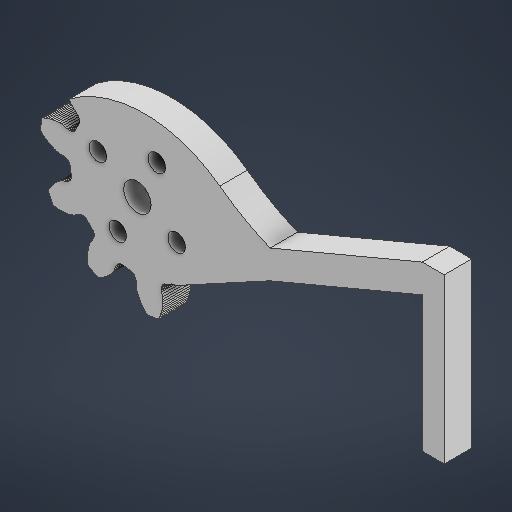
# Autodesk Inventor part: писюн
Saved by Autodesk Inventor 2025 (Build 290162000, 162)
## iProperties
Created: 2024-12-28
Part Number: писюн
Material: Типовые
Document SubType Name: Modeling
Designer: Phantom
Density: 1 g/cm^3
Appearance: По умолчанию
Author: Phantom
Autodesk Inventor part; units mm, degrees
(part 1 of 2)
ref_plane "YZ Plane" through (0, 0, 0) normal (1, 0, 0) x (0, 1, 0)
ref_plane "XZ Plane" through (0, 0, 0) normal (0, 1, 0) x (-1, 0, 0)
ref_plane "XY Plane" through (0, 0, 0) normal (0, 0, 1) x (1, 0, 0)
sketch "Эскиз1" plane through (0, 0, 0) normal (0, 0, 1) x (1, 0, 0)
  arc A0 (25.3405, 9.161) -> (8.4316, -5.5092) centre (48.8211, -34.9827) ccw
  arc A1 (16.1963, 14.3431) -> (25.3405, 9.161) centre (40.8164, 47.1281) ccw
  arc A2 (16.1963, 14.3431) -> (-11.1891, 14.3431) centre (2.5036, -3.8906) ccw
  line L0 (-11.1891, 14.3431) -> (-11.0924, 14.1698)
  line L1 (-11.0924, 14.1698) -> (-10.8798, 13.8428)
  line L2 (-10.8798, 13.8428) -> (-10.6476, 13.5415)
  line L3 (-10.6476, 13.5415) -> (-10.3902, 13.2744)
  line L4 (-10.3902, 13.2744) -> (-10.0964, 13.0589)
  line L5 (-10.0964, 13.0589) -> (-9.8198, 12.8188)
  line L6 (-9.8198, 12.8188) -> (-9.6918, 12.6838)
  line L7 (-9.6918, 12.6838) -> (-9.5723, 12.5363)
  line L8 (-9.5723, 12.5363) -> (-9.4633, 12.3731)
  line L9 (-9.4633, 12.3731) -> (-9.3681, 12.1883)
  line L10 (-9.3681, 12.1883) -> (-9.3278, 12.0845)
  line L11 (-9.3278, 12.0845) -> (-9.2943, 11.9695)
  line L12 (-9.2943, 11.9695) -> (-9.2712, 11.8376)
  line L13 (-9.2712, 11.8376) -> (-9.2668, 11.6743)
  line L14 (-9.2668, 11.6743) -> (-9.3696, 11.329)
  line L15 (-9.3696, 11.329) -> (-9.7265, 10.6764)
  line L16 (-9.7265, 10.6764) -> (-10.0432, 10.0032)
  line L17 (-10.0432, 10.0032) -> (-10.2615, 9.7167)
  line L18 (-10.2615, 9.7167) -> (-10.3959, 9.6239)
  line L19 (-10.3959, 9.6239) -> (-10.5161, 9.5649)
  line L20 (-10.5161, 9.5649) -> (-10.6287, 9.5241)
  line L21 (-10.6287, 9.5241) -> (-10.7364, 9.4955)
  line L22 (-10.7364, 9.4955) -> (-10.9417, 9.4634)
  line L23 (-10.9417, 9.4634) -> (-11.1379, 9.4552)
  line L24 (-11.1379, 9.4552) -> (-11.3274, 9.4648)
  line L25 (-11.3274, 9.4648) -> (-11.5119, 9.4885)
  line L26 (-11.5119, 9.4885) -> (-11.8689, 9.5704)
  line L27 (-11.8689, 9.5704) -> (-12.2162, 9.6807)
  line L28 (-12.2162, 9.6807) -> (-12.5837, 9.731)
  line L29 (-12.5837, 9.731) -> (-12.964, 9.741)
  line L30 (-12.964, 9.741) -> (-13.3534, 9.7199)
  line L31 (-13.3534, 9.7199) -> (-13.7498, 9.6714)
  line L32 (-13.7498, 9.6714) -> (-14.1519, 9.5976)
  line L33 (-14.1519, 9.5976) -> (-14.5586, 9.4998)
  line L34 (-14.5586, 9.4998) -> (-14.9687, 9.3787)
  line L35 (-14.9687, 9.3787) -> (-15.3815, 9.2349)
  line L36 (-15.3815, 9.2349) -> (-15.796, 9.069)
  line L37 (-15.796, 9.069) -> (-16.1075, 8.9301)
  line L38 (-16.1075, 8.9301) -> (-16.4414, 6.8067)
  line L39 (-16.4414, 6.8067) -> (-16.1875, 6.579)
  line L40 (-16.1875, 6.579) -> (-15.8439, 6.2938)
  line L41 (-15.8439, 6.2938) -> (-15.4952, 6.0303)
  line L42 (-15.4952, 6.0303) -> (-15.142, 5.7892)
  line L43 (-15.142, 5.7892) -> (-14.785, 5.5713)
  line L44 (-14.785, 5.5713) -> (-14.425, 5.3776)
  line L45 (-14.425, 5.3776) -> (-14.0625, 5.2099)
  line L46 (-14.0625, 5.2099) -> (-13.6984, 5.0703)
  line L47 (-13.6984, 5.0703) -> (-13.3334, 4.963)
  line L48 (-13.3334, 4.963) -> (-12.9682, 4.8982)
  line L49 (-12.9682, 4.8982) -> (-12.6038, 4.8965)
  line L50 (-12.6038, 4.8965) -> (-12.2389, 4.8649)
  line L51 (-12.2389, 4.8649) -> (-12.056, 4.8309)
  line L52 (-12.056, 4.8309) -> (-11.8727, 4.7818)
  line L53 (-11.8727, 4.7818) -> (-11.6885, 4.7139)
  line L54 (-11.6885, 4.7139) -> (-11.5029, 4.6203)
  line L55 (-11.5029, 4.6203) -> (-11.4093, 4.56)
  line L56 (-11.4093, 4.56) -> (-11.3146, 4.4866)
  line L57 (-11.3146, 4.4866) -> (-11.2183, 4.3936)
  line L58 (-11.2183, 4.3936) -> (-11.1188, 4.264)
  line L59 (-11.1188, 4.264) -> (-10.999, 3.9243)
  line L60 (-10.999, 3.9243) -> (-10.9042, 3.1865)
  line L61 (-10.9042, 3.1865) -> (-10.7647, 2.4558)
  line L62 (-10.7647, 2.4558) -> (-10.7729, 2.0956)
  line L63 (-10.7729, 2.0956) -> (-10.8272, 1.9416)
  line L64 (-10.8272, 1.9416) -> (-10.8897, 1.8232)
  line L65 (-10.8897, 1.8232) -> (-10.9568, 1.724)
  line L66 (-10.9568, 1.724) -> (-11.0271, 1.6375)
  line L67 (-11.0271, 1.6375) -> (-11.1743, 1.4909)
  line L68 (-11.1743, 1.4909) -> (-11.3282, 1.369)
  line L69 (-11.3282, 1.369) -> (-11.4872, 1.2653)
  line L70 (-11.4872, 1.2653) -> (-11.6504, 1.1761)
  line L71 (-11.6504, 1.1761) -> (-11.9874, 1.0325)
  line L72 (-11.9874, 1.0325) -> (-12.3332, 0.9175)
  line L73 (-12.3332, 0.9175) -> (-12.66, 0.7423)
  line L74 (-12.66, 0.7423) -> (-12.9736, 0.5268)
  line L75 (-12.9736, 0.5268) -> (-13.2762, 0.2808)
  line L76 (-13.2762, 0.2808) -> (-13.5684, 0.0086)
  line L77 (-13.5684, 0.0086) -> (-13.8504, -0.2874)
  line L78 (-13.8504, -0.2874) -> (-14.1218, -0.6056)
  line L79 (-14.1218, -0.6056) -> (-14.3824, -0.9447)
  line L80 (-14.3824, -0.9447) -> (-14.6319, -1.3036)
  line L81 (-14.6319, -1.3036) -> (-14.8697, -1.6815)
  line L82 (-14.8697, -1.6815) -> (-15.0401, -1.9769)
  line L83 (-15.0401, -1.9769) -> (-14.0621, -3.891)
  line L84 (-14.0621, -3.891) -> (-13.7228, -3.9261)
  line L85 (-13.7228, -3.9261) -> (-13.2773, -3.9548)
  line L86 (-13.2773, -3.9548) -> (-12.8403, -3.963)
  line L87 (-12.8403, -3.963) -> (-12.4128, -3.9505)
  line L88 (-12.4128, -3.9505) -> (-11.9959, -3.917)
  line L89 (-11.9959, -3.917) -> (-11.5908, -3.862)
  line L90 (-11.5908, -3.862) -> (-11.199, -3.7847)
  line L91 (-11.199, -3.7847) -> (-10.8224, -3.6836)
  line L92 (-10.8224, -3.6836) -> (-10.464, -3.5558)
  line L93 (-10.464, -3.5558) -> (-10.1304, -3.3936)
  line L94 (-10.1304, -3.3936) -> (-9.8347, -3.1808)
  line L95 (-9.8347, -3.1808) -> (-9.5209, -2.9918)
  line L96 (-9.5209, -2.9918) -> (-9.353, -2.9118)
  line L97 (-9.353, -2.9118) -> (-9.1758, -2.8438)
  line L98 (-9.1758, -2.8438) -> (-8.9868, -2.7905)
  line L99 (-8.9868, -2.7905) -> (-8.7817, -2.7571)
  line L100 (-8.7817, -2.7571) -> (-8.6705, -2.7509)
  line L101 (-8.6705, -2.7509) -> (-8.5508, -2.7546)
  line L102 (-8.5508, -2.7546) -> (-8.4182, -2.7733)
  line L103 (-8.4182, -2.7733) -> (-8.2615, -2.8196)
  line L104 (-8.2615, -2.8196) -> (-7.9649, -3.024)
  line L105 (-7.9649, -3.024) -> (-7.4545, -3.5652)
  line L106 (-7.4545, -3.5652) -> (-6.9122, -4.0744)
  line L107 (-6.9122, -4.0744) -> (-6.7071, -4.3705)
  line L108 (-6.7071, -4.3705) -> (-6.6604, -4.5271)
  line L109 (-6.6604, -4.5271) -> (-6.6415, -4.6596)
  line L110 (-6.6415, -4.6596) -> (-6.6374, -4.7793)
  line L111 (-6.6374, -4.7793) -> (-6.6435, -4.8906)
  line L112 (-6.6435, -4.8906) -> (-6.6764, -5.0958)
  line L113 (-6.6764, -5.0958) -> (-6.7292, -5.2848)
  line L114 (-6.7292, -5.2848) -> (-6.7969, -5.4622)
  line L115 (-6.7969, -5.4622) -> (-6.8765, -5.6303)
  line L116 (-6.8765, -5.6303) -> (-7.0647, -5.9445)
  line L117 (-7.0647, -5.9445) -> (-7.2769, -6.2407)
  line L118 (-7.2769, -6.2407) -> (-7.4384, -6.5746)
  line L119 (-7.4384, -6.5746) -> (-7.5654, -6.9333)
  line L120 (-7.5654, -6.9333) -> (-7.6656, -7.3102)
  line L121 (-7.6656, -7.3102) -> (-7.742, -7.7022)
  line L122 (-7.742, -7.7022) -> (-7.7961, -8.1074)
  line L123 (-7.7961, -8.1074) -> (-7.8287, -8.5243)
  line L124 (-7.8287, -8.5243) -> (-7.8403, -8.9518)
  line L125 (-7.8403, -8.9518) -> (-7.8311, -9.3888)
  line L126 (-7.8311, -9.3888) -> (-7.8013, -9.8343)
  line L127 (-7.8013, -9.8343) -> (-7.7656, -10.1735)
  line L128 (-7.7656, -10.1735) -> (-5.8492, -11.1472)
  line L129 (-5.8492, -11.1472) -> (-5.5542, -10.9761)
  line L130 (-5.5542, -10.9761) -> (-5.1768, -10.7375)
  line L131 (-5.1768, -10.7375) -> (-4.8185, -10.4872)
  line L132 (-4.8185, -10.4872) -> (-4.48, -10.2258)
  line L133 (-4.48, -10.2258) -> (-4.1624, -9.9537)
  line L134 (-4.1624, -9.9537) -> (-3.867, -9.6711)
  line L135 (-3.867, -9.6711) -> (-3.5955, -9.3782)
  line L136 (-3.5955, -9.3782) -> (-3.3502, -9.0751)
  line L137 (-3.3502, -9.0751) -> (-3.1354, -8.7611)
  line L138 (-3.1354, -8.7611) -> (-2.9609, -8.4338)
  line L139 (-2.9609, -8.4338) -> (-2.8467, -8.0877)
  line L140 (-2.8467, -8.0877) -> (-2.7039, -7.7505)
  line L141 (-2.7039, -7.7505) -> (-2.615, -7.5871)
  line L142 (-2.615, -7.5871) -> (-2.5117, -7.4278)
  line L143 (-2.5117, -7.4278) -> (-2.3901, -7.2737)
  line L144 (-2.3901, -7.2737) -> (-2.2438, -7.1261)
  line L145 (-2.2438, -7.1261) -> (-2.1575, -7.0556)
  line L146 (-2.1575, -7.0556) -> (-2.0585, -6.9883)
  line L147 (-2.0585, -6.9883) -> (-1.9402, -6.9255)
  line L148 (-1.9402, -6.9255) -> (-1.7863, -6.8709)
  line L149 (-1.7863, -6.8709) -> (-1.4262, -6.8619)
  line L150 (-1.4262, -6.8619) -> (-0.6951, -6.9997)
  line L151 (-0.6951, -6.9997) -> (0.0429, -7.0929)
  line L152 (0.0429, -7.0929) -> (0.3829, -7.2119)
  line L153 (0.3829, -7.2119) -> (0.5127, -7.3112)
  line L154 (0.5127, -7.3112) -> (0.6059, -7.4072)
  line L155 (0.6059, -7.4072) -> (0.6795, -7.5017)
  line L156 (0.6795, -7.5017) -> (0.74, -7.5953)
  line L157 (0.74, -7.5953) -> (0.834, -7.7806)
  line L158 (0.834, -7.7806) -> (0.9024, -7.9646)
  line L159 (0.9024, -7.9646) -> (0.9519, -8.1479)
  line L160 (0.9519, -8.1479) -> (0.9863, -8.3307)
  line L161 (0.9863, -8.3307) -> (1.0187, -8.6955)
  line L162 (1.0187, -8.6955) -> (1.0212, -9.0599)
  line L163 (1.0212, -9.0599) -> (1.0869, -9.4249)
  line L164 (1.0869, -9.4249) -> (1.1949, -9.7897)
  line L165 (1.1949, -9.7897) -> (1.3353, -10.1535)
  line L166 (1.3353, -10.1535) -> (1.5039, -10.5156)
  line L167 (1.5039, -10.5156) -> (1.6983, -10.8752)
  line L168 (1.6983, -10.8752) -> (1.9171, -11.2317)
  line L169 (1.9171, -11.2317) -> (2.159, -11.5843)
  line L170 (2.159, -11.5843) -> (2.4233, -11.9325)
  line L171 (2.4233, -11.9325) -> (2.7092, -12.2754)
  line L172 (2.7092, -12.2754) -> (2.9375, -12.5288)
  line L173 (2.9375, -12.5288) -> (5.0602, -12.1901)
  line L174 (5.0602, -12.1901) -> (5.1983, -11.8783)
  line L175 (5.1983, -11.8783) -> (5.3633, -11.4634)
  line L176 (5.3633, -11.4634) -> (5.5062, -11.0504)
  line L177 (5.5062, -11.0504) -> (5.6263, -10.6399)
  line L178 (5.6263, -10.6399) -> (5.7233, -10.2331)
  line L179 (5.7233, -10.2331) -> (5.7962, -9.8308)
  line L180 (5.7962, -9.8308) -> (5.8437, -9.4343)
  line L181 (5.8437, -9.4343) -> (5.864, -9.0449)
  line L182 (5.864, -9.0449) -> (5.8532, -8.6645)
  line L183 (5.8532, -8.6645) -> (5.802, -8.2972)
  line L184 (5.802, -8.2972) -> (5.691, -7.9502)
  line L185 (5.691, -7.9502) -> (5.6083, -7.5933)
  line L186 (5.6083, -7.5933) -> (5.5841, -7.4089)
  line L187 (5.5841, -7.4089) -> (5.5741, -7.2193)
  line L188 (5.5741, -7.2193) -> (5.5818, -7.0232)
  line L189 (5.5818, -7.0232) -> (5.6135, -6.8178)
  line L190 (5.6135, -6.8178) -> (5.6419, -6.7101)
  line L191 (5.6419, -6.7101) -> (5.6824, -6.5974)
  line L192 (5.6824, -6.5974) -> (5.7412, -6.4771)
  line L193 (5.7412, -6.4771) -> (5.8336, -6.3424)
  line L194 (5.8336, -6.3424) -> (6.1197, -6.1235)
  line L195 (6.1197, -6.1235) -> (6.7921, -5.8052)
  line L196 (6.7921, -5.8052) -> (7.444, -5.4468)
  line L197 (7.444, -5.4468) -> (7.789, -5.3433)
  line L198 (7.789, -5.3433) -> (7.9523, -5.3473)
  line L199 (7.9523, -5.3473) -> (8.0842, -5.3702)
  line L200 (8.0842, -5.3702) -> (8.1993, -5.4034)
  line L201 (8.1993, -5.4034) -> (8.3032, -5.4435)
  line L202 (8.3032, -5.4435) -> (8.4316, -5.5092)
  circle A3 centre (-5.9559, 8.675) radius 1.6
  circle A4 centre (-2.3455, -2.0471) radius 1.6
  circle A5 centre (8.3767, 1.5633) radius 1.6
  circle A6 centre (4.7663, 12.2855) radius 1.6
  circle A7 centre (1.2104, 5.1192) radius 2.5
  point P0 (0, 0)
  point P1 (-20.9679, -17.3277)
  constraints: 406 end point, 8 centre point, 6 point on circle
extrude "Выдавливание1" add sketch "Эскиз1" along normal blind 5
sketch "Эскиз2" plane through (0, 0, 0) normal (0, 0, -1) x (-1, 0, 0)
  line L0 (-8.3032, -5.4435) -> (-8.4316, -5.5092) projected
  line L1 (-8.4316, -5.5092) -> (-25.3405, -5.5092)
  line L2 (11.1891, 14.3431) -> (11.0924, 14.1698) projected
  arc A0 (11.1891, 14.3431) -> (-16.1963, 14.3431) centre (-2.5036, -3.8906) ccw projected
  arc A1 (-25.3405, 9.161) -> (-16.1963, 14.3431) centre (-40.8164, 47.1281) ccw projected
  arc A2 (-8.4316, -5.5092) -> (-25.3405, 9.161) centre (-48.8211, -34.9827) ccw projected
  line L3 (-8.3032, -5.4435) -> (-8.4316, -5.5092) projected
  line L4 (-8.1993, -5.4034) -> (-8.3032, -5.4435) projected
  line L5 (-8.0842, -5.3702) -> (-8.1993, -5.4034) projected
  line L6 (-7.9523, -5.3473) -> (-8.0842, -5.3702) projected
  line L7 (-7.789, -5.3433) -> (-7.9523, -5.3473) projected
  line L8 (-7.444, -5.4468) -> (-7.789, -5.3433) projected
  line L9 (-6.7921, -5.8052) -> (-7.444, -5.4468) projected
  line L10 (-6.1197, -6.1235) -> (-6.7921, -5.8052) projected
  line L11 (-5.8336, -6.3424) -> (-6.1197, -6.1235) projected
  line L12 (-5.7412, -6.4771) -> (-5.8336, -6.3424) projected
  line L13 (-5.6824, -6.5974) -> (-5.7412, -6.4771) projected
  line L14 (-5.6419, -6.7101) -> (-5.6824, -6.5974) projected
  line L15 (-5.6135, -6.8178) -> (-5.6419, -6.7101) projected
  line L16 (-5.5818, -7.0232) -> (-5.6135, -6.8178) projected
  line L17 (-5.5741, -7.2193) -> (-5.5818, -7.0232) projected
  line L18 (-5.5841, -7.4089) -> (-5.5741, -7.2193) projected
  line L19 (-5.6083, -7.5933) -> (-5.5841, -7.4089) projected
  line L20 (-5.691, -7.9502) -> (-5.6083, -7.5933) projected
  line L21 (-5.802, -8.2972) -> (-5.691, -7.9502) projected
  line L22 (-5.8532, -8.6645) -> (-5.802, -8.2972) projected
  line L23 (-5.864, -9.0449) -> (-5.8532, -8.6645) projected
  line L24 (-5.8437, -9.4343) -> (-5.864, -9.0449) projected
  line L25 (-5.7962, -9.8308) -> (-5.8437, -9.4343) projected
  line L26 (-5.7233, -10.2331) -> (-5.7962, -9.8308) projected
  line L27 (-5.6263, -10.6399) -> (-5.7233, -10.2331) projected
  line L28 (-5.5062, -11.0504) -> (-5.6263, -10.6399) projected
  line L29 (-5.3633, -11.4634) -> (-5.5062, -11.0504) projected
  line L30 (-5.1983, -11.8783) -> (-5.3633, -11.4634) projected
  line L31 (-5.0602, -12.1901) -> (-5.1983, -11.8783) projected
  line L32 (-2.9375, -12.5288) -> (-5.0602, -12.1901) projected
  line L33 (-2.7092, -12.2754) -> (-2.9375, -12.5288) projected
  line L34 (-2.4233, -11.9325) -> (-2.7092, -12.2754) projected
  line L35 (-2.159, -11.5843) -> (-2.4233, -11.9325) projected
  line L36 (-1.9171, -11.2317) -> (-2.159, -11.5843) projected
  line L37 (-1.6983, -10.8752) -> (-1.9171, -11.2317) projected
  line L38 (-1.5039, -10.5156) -> (-1.6983, -10.8752) projected
  line L39 (-1.3353, -10.1535) -> (-1.5039, -10.5156) projected
  line L40 (-1.1949, -9.7897) -> (-1.3353, -10.1535) projected
  line L41 (-1.0869, -9.4249) -> (-1.1949, -9.7897) projected
  line L42 (-1.0212, -9.0599) -> (-1.0869, -9.4249) projected
  line L43 (-1.0187, -8.6955) -> (-1.0212, -9.0599) projected
  line L44 (-0.9863, -8.3307) -> (-1.0187, -8.6955) projected
  line L45 (-0.9519, -8.1479) -> (-0.9863, -8.3307) projected
  line L46 (-0.9024, -7.9646) -> (-0.9519, -8.1479) projected
  line L47 (-0.834, -7.7806) -> (-0.9024, -7.9646) projected
  line L48 (-0.74, -7.5953) -> (-0.834, -7.7806) projected
  line L49 (-0.6795, -7.5017) -> (-0.74, -7.5953) projected
  line L50 (-0.6059, -7.4072) -> (-0.6795, -7.5017) projected
  line L51 (-0.5127, -7.3112) -> (-0.6059, -7.4072) projected
  line L52 (-0.3829, -7.2119) -> (-0.5127, -7.3112) projected
  line L53 (-0.0429, -7.0929) -> (-0.3829, -7.2119) projected
  line L54 (0.6951, -6.9997) -> (-0.0429, -7.0929) projected
  line L55 (1.4262, -6.8619) -> (0.6951, -6.9997) projected
  line L56 (1.7863, -6.8709) -> (1.4262, -6.8619) projected
  line L57 (1.9402, -6.9255) -> (1.7863, -6.8709) projected
  line L58 (2.0585, -6.9883) -> (1.9402, -6.9255) projected
  line L59 (2.1575, -7.0556) -> (2.0585, -6.9883) projected
  line L60 (2.2438, -7.1261) -> (2.1575, -7.0556) projected
  line L61 (2.3901, -7.2737) -> (2.2438, -7.1261) projected
  line L62 (2.5117, -7.4278) -> (2.3901, -7.2737) projected
  line L63 (2.615, -7.5871) -> (2.5117, -7.4278) projected
  line L64 (2.7039, -7.7505) -> (2.615, -7.5871) projected
  line L65 (2.8467, -8.0877) -> (2.7039, -7.7505) projected
  line L66 (2.9609, -8.4338) -> (2.8467, -8.0877) projected
  line L67 (3.1354, -8.7611) -> (2.9609, -8.4338) projected
  line L68 (3.3502, -9.0751) -> (3.1354, -8.7611) projected
  line L69 (3.5955, -9.3782) -> (3.3502, -9.0751) projected
  line L70 (3.867, -9.6711) -> (3.5955, -9.3782) projected
  line L71 (4.1624, -9.9537) -> (3.867, -9.6711) projected
  line L72 (4.48, -10.2258) -> (4.1624, -9.9537) projected
  line L73 (4.8185, -10.4872) -> (4.48, -10.2258) projected
  line L74 (5.1768, -10.7375) -> (4.8185, -10.4872) projected
  line L75 (5.5542, -10.9761) -> (5.1768, -10.7375) projected
  line L76 (5.8492, -11.1472) -> (5.5542, -10.9761) projected
  line L77 (7.7656, -10.1735) -> (5.8492, -11.1472) projected
  line L78 (7.8013, -9.8343) -> (7.7656, -10.1735) projected
  line L79 (7.8311, -9.3888) -> (7.8013, -9.8343) projected
  line L80 (7.8403, -8.9518) -> (7.8311, -9.3888) projected
  line L81 (7.8287, -8.5243) -> (7.8403, -8.9518) projected
  line L82 (7.7961, -8.1074) -> (7.8287, -8.5243) projected
  line L83 (7.742, -7.7022) -> (7.7961, -8.1074) projected
  line L84 (7.6656, -7.3102) -> (7.742, -7.7022) projected
  line L85 (7.5654, -6.9333) -> (7.6656, -7.3102) projected
  line L86 (7.4384, -6.5746) -> (7.5654, -6.9333) projected
  line L87 (7.2769, -6.2407) -> (7.4384, -6.5746) projected
  line L88 (7.0647, -5.9445) -> (7.2769, -6.2407) projected
  line L89 (6.8765, -5.6303) -> (7.0647, -5.9445) projected
  line L90 (6.7969, -5.4622) -> (6.8765, -5.6303) projected
  line L91 (6.7292, -5.2848) -> (6.7969, -5.4622) projected
  line L92 (6.6764, -5.0958) -> (6.7292, -5.2848) projected
  line L93 (6.6435, -4.8906) -> (6.6764, -5.0958) projected
  line L94 (6.6374, -4.7793) -> (6.6435, -4.8906) projected
  line L95 (6.6415, -4.6596) -> (6.6374, -4.7793) projected
  line L96 (6.6604, -4.5271) -> (6.6415, -4.6596) projected
  line L97 (6.7071, -4.3705) -> (6.6604, -4.5271) projected
  line L98 (6.9122, -4.0744) -> (6.7071, -4.3705) projected
  line L99 (7.4545, -3.5652) -> (6.9122, -4.0744) projected
  line L100 (7.9649, -3.024) -> (7.4545, -3.5652) projected
  line L101 (8.2615, -2.8196) -> (7.9649, -3.024) projected
  line L102 (8.4182, -2.7733) -> (8.2615, -2.8196) projected
  line L103 (8.5508, -2.7546) -> (8.4182, -2.7733) projected
  line L104 (8.6705, -2.7509) -> (8.5508, -2.7546) projected
  line L105 (8.7817, -2.7571) -> (8.6705, -2.7509) projected
  line L106 (8.9868, -2.7905) -> (8.7817, -2.7571) projected
  line L107 (9.1758, -2.8438) -> (8.9868, -2.7905) projected
  line L108 (9.353, -2.9118) -> (9.1758, -2.8438) projected
  line L109 (9.5209, -2.9918) -> (9.353, -2.9118) projected
  line L110 (9.8347, -3.1808) -> (9.5209, -2.9918) projected
  line L111 (10.1304, -3.3936) -> (9.8347, -3.1808) projected
  line L112 (10.464, -3.5558) -> (10.1304, -3.3936) projected
  line L113 (10.8224, -3.6836) -> (10.464, -3.5558) projected
  line L114 (11.199, -3.7847) -> (10.8224, -3.6836) projected
  line L115 (11.5908, -3.862) -> (11.199, -3.7847) projected
  line L116 (11.9959, -3.917) -> (11.5908, -3.862) projected
  line L117 (12.4128, -3.9505) -> (11.9959, -3.917) projected
  line L118 (12.8403, -3.963) -> (12.4128, -3.9505) projected
  line L119 (13.2773, -3.9548) -> (12.8403, -3.963) projected
  line L120 (13.7228, -3.9261) -> (13.2773, -3.9548) projected
  line L121 (14.0621, -3.891) -> (13.7228, -3.9261) projected
  line L122 (15.0401, -1.9769) -> (14.0621, -3.891) projected
  line L123 (14.8697, -1.6815) -> (15.0401, -1.9769) projected
  line L124 (14.6319, -1.3036) -> (14.8697, -1.6815) projected
  line L125 (14.3824, -0.9447) -> (14.6319, -1.3036) projected
  line L126 (14.1218, -0.6056) -> (14.3824, -0.9447) projected
  line L127 (13.8504, -0.2874) -> (14.1218, -0.6056) projected
  line L128 (13.5684, 0.0086) -> (13.8504, -0.2874) projected
  line L129 (13.2762, 0.2808) -> (13.5684, 0.0086) projected
  line L130 (12.9736, 0.5268) -> (13.2762, 0.2808) projected
  line L131 (12.66, 0.7423) -> (12.9736, 0.5268) projected
  line L132 (12.3332, 0.9175) -> (12.66, 0.7423) projected
  line L133 (11.9874, 1.0325) -> (12.3332, 0.9175) projected
  line L134 (11.6504, 1.1761) -> (11.9874, 1.0325) projected
  line L135 (11.4872, 1.2653) -> (11.6504, 1.1761) projected
  line L136 (11.3282, 1.369) -> (11.4872, 1.2653) projected
  line L137 (11.1743, 1.4909) -> (11.3282, 1.369) projected
  line L138 (11.0271, 1.6375) -> (11.1743, 1.4909) projected
  line L139 (10.9568, 1.724) -> (11.0271, 1.6375) projected
  line L140 (10.8897, 1.8232) -> (10.9568, 1.724) projected
  line L141 (10.8272, 1.9416) -> (10.8897, 1.8232) projected
  line L142 (10.7729, 2.0956) -> (10.8272, 1.9416) projected
  line L143 (10.7647, 2.4558) -> (10.7729, 2.0956) projected
  line L144 (10.9042, 3.1865) -> (10.7647, 2.4558) projected
  line L145 (10.999, 3.9243) -> (10.9042, 3.1865) projected
  line L146 (11.1188, 4.264) -> (10.999, 3.9243) projected
  line L147 (11.2183, 4.3936) -> (11.1188, 4.264) projected
  line L148 (11.3146, 4.4866) -> (11.2183, 4.3936) projected
  line L149 (11.4093, 4.56) -> (11.3146, 4.4866) projected
  line L150 (11.5029, 4.6203) -> (11.4093, 4.56) projected
  line L151 (11.6885, 4.7139) -> (11.5029, 4.6203) projected
  line L152 (11.8727, 4.7818) -> (11.6885, 4.7139) projected
  line L153 (12.056, 4.8309) -> (11.8727, 4.7818) projected
  line L154 (12.2389, 4.8649) -> (12.056, 4.8309) projected
  line L155 (12.6038, 4.8965) -> (12.2389, 4.8649) projected
  line L156 (12.9682, 4.8982) -> (12.6038, 4.8965) projected
  line L157 (13.3334, 4.963) -> (12.9682, 4.8982) projected
  line L158 (13.6984, 5.0703) -> (13.3334, 4.963) projected
  line L159 (14.0625, 5.2099) -> (13.6984, 5.0703) projected
  line L160 (14.425, 5.3776) -> (14.0625, 5.2099) projected
  line L161 (14.785, 5.5713) -> (14.425, 5.3776) projected
  line L162 (15.142, 5.7892) -> (14.785, 5.5713) projected
  line L163 (15.4952, 6.0303) -> (15.142, 5.7892) projected
  line L164 (15.8439, 6.2938) -> (15.4952, 6.0303) projected
  line L165 (16.1875, 6.579) -> (15.8439, 6.2938) projected
  line L166 (16.4414, 6.8067) -> (16.1875, 6.579) projected
  line L167 (16.1075, 8.9301) -> (16.4414, 6.8067) projected
  line L168 (15.796, 9.069) -> (16.1075, 8.9301) projected
  line L169 (15.3815, 9.2349) -> (15.796, 9.069) projected
  line L170 (14.9687, 9.3787) -> (15.3815, 9.2349) projected
  line L171 (14.5586, 9.4998) -> (14.9687, 9.3787) projected
  line L172 (14.1519, 9.5976) -> (14.5586, 9.4998) projected
  line L173 (13.7498, 9.6714) -> (14.1519, 9.5976) projected
  line L174 (13.3534, 9.7199) -> (13.7498, 9.6714) projected
  line L175 (12.964, 9.741) -> (13.3534, 9.7199) projected
  line L176 (12.5837, 9.731) -> (12.964, 9.741) projected
  line L177 (12.2162, 9.6807) -> (12.5837, 9.731) projected
  line L178 (11.8689, 9.5704) -> (12.2162, 9.6807) projected
  line L179 (11.5119, 9.4885) -> (11.8689, 9.5704) projected
  line L180 (11.3274, 9.4648) -> (11.5119, 9.4885) projected
  line L181 (11.1379, 9.4552) -> (11.3274, 9.4648) projected
  line L182 (10.9417, 9.4634) -> (11.1379, 9.4552) projected
  line L183 (10.7364, 9.4955) -> (10.9417, 9.4634) projected
  line L184 (10.6287, 9.5241) -> (10.7364, 9.4955) projected
  line L185 (10.5161, 9.5649) -> (10.6287, 9.5241) projected
  line L186 (10.3959, 9.6239) -> (10.5161, 9.5649) projected
  line L187 (10.2615, 9.7167) -> (10.3959, 9.6239) projected
  line L188 (10.0432, 10.0032) -> (10.2615, 9.7167) projected
  line L189 (9.7265, 10.6764) -> (10.0432, 10.0032) projected
  line L190 (9.3696, 11.329) -> (9.7265, 10.6764) projected
  line L191 (9.2668, 11.6743) -> (9.3696, 11.329) projected
  line L192 (9.2712, 11.8376) -> (9.2668, 11.6743) projected
  line L193 (9.2943, 11.9695) -> (9.2712, 11.8376) projected
  line L194 (9.3278, 12.0845) -> (9.2943, 11.9695) projected
  line L195 (9.3681, 12.1883) -> (9.3278, 12.0845) projected
  line L196 (9.4633, 12.3731) -> (9.3681, 12.1883) projected
  line L197 (9.5723, 12.5363) -> (9.4633, 12.3731) projected
  line L198 (9.6918, 12.6838) -> (9.5723, 12.5363) projected
  line L199 (9.8198, 12.8188) -> (9.6918, 12.6838) projected
  line L200 (10.0964, 13.0589) -> (9.8198, 12.8188) projected
  line L201 (10.3902, 13.2744) -> (10.0964, 13.0589) projected
  line L202 (10.6476, 13.5415) -> (10.3902, 13.2744) projected
  line L203 (10.8798, 13.8428) -> (10.6476, 13.5415) projected
  line L204 (11.0924, 14.1698) -> (10.8798, 13.8428) projected
  circle A3 centre (-8.3767, 1.5633) radius 1.6 projected
  circle A4 centre (2.3455, -2.0471) radius 1.6 projected
  circle A5 centre (5.9559, 8.675) radius 1.6 projected
  circle A6 centre (-4.7663, 12.2855) radius 1.6 projected
  circle A7 centre (-1.2104, 5.1192) radius 2.5 projected
  line L205 (-25.3405, 9.161) -> (-25.3405, -5.5092)
  point P0 (0, 0)
  constraints: 4 end point, 1 horizontal, 1 perpendicular
extrude "Выдавливание2" add sketch "Эскиз2" against normal up to surface (5 mm away) contours L1 L205 A2
sketch "Эскиз3" plane through (0, 0, 0) normal (0, 0, -1) x (-1, 0, 0)
  line L0 (-25.3405, 9.161) -> (-25.3405, -5.5092) projected
  line L1 (-25.3405, 9.161) -> (-53, 20.778)
  line L2 (-53, 20.778) -> (-76.2555, 1.8259)
  line L3 (-76.2555, 1.8259) -> (-73.7286, -1.2748)
  line L4 (-73.7286, -1.2748) -> (-53, 15.6179)
  line L5 (-53, 15.6179) -> (-25.3405, 4.0009)
  line L6 (11.1891, 14.3431) -> (11.0924, 14.1698) projected
  arc A0 (11.1891, 14.3431) -> (-16.1963, 14.3431) centre (-2.5036, -3.8906) ccw projected
  arc A1 (-25.3405, 9.161) -> (-16.1963, 14.3431) centre (-40.8164, 47.1281) ccw projected
  line L7 (-25.3405, 9.161) -> (-25.3405, -5.5092) projected
  line L8 (-25.3405, -5.5092) -> (-8.4316, -5.5092) projected
  line L9 (-8.3032, -5.4435) -> (-8.4316, -5.5092) projected
  line L10 (-8.1993, -5.4034) -> (-8.3032, -5.4435) projected
  line L11 (-8.0842, -5.3702) -> (-8.1993, -5.4034) projected
  line L12 (-7.9523, -5.3473) -> (-8.0842, -5.3702) projected
  line L13 (-7.789, -5.3433) -> (-7.9523, -5.3473) projected
  line L14 (-7.444, -5.4468) -> (-7.789, -5.3433) projected
  line L15 (-6.7921, -5.8052) -> (-7.444, -5.4468) projected
  line L16 (-6.1197, -6.1235) -> (-6.7921, -5.8052) projected
  line L17 (-5.8336, -6.3424) -> (-6.1197, -6.1235) projected
  line L18 (-5.7412, -6.4771) -> (-5.8336, -6.3424) projected
  line L19 (-5.6824, -6.5974) -> (-5.7412, -6.4771) projected
  line L20 (-5.6419, -6.7101) -> (-5.6824, -6.5974) projected
  line L21 (-5.6135, -6.8178) -> (-5.6419, -6.7101) projected
  line L22 (-5.5818, -7.0232) -> (-5.6135, -6.8178) projected
  line L23 (-5.5741, -7.2193) -> (-5.5818, -7.0232) projected
  line L24 (-5.5841, -7.4089) -> (-5.5741, -7.2193) projected
  line L25 (-5.6083, -7.5933) -> (-5.5841, -7.4089) projected
  line L26 (-5.691, -7.9502) -> (-5.6083, -7.5933) projected
  line L27 (-5.802, -8.2972) -> (-5.691, -7.9502) projected
  line L28 (-5.8532, -8.6645) -> (-5.802, -8.2972) projected
  line L29 (-5.864, -9.0449) -> (-5.8532, -8.6645) projected
  line L30 (-5.8437, -9.4343) -> (-5.864, -9.0449) projected
  line L31 (-5.7962, -9.8308) -> (-5.8437, -9.4343) projected
  line L32 (-5.7233, -10.2331) -> (-5.7962, -9.8308) projected
  line L33 (-5.6263, -10.6399) -> (-5.7233, -10.2331) projected
  line L34 (-5.5062, -11.0504) -> (-5.6263, -10.6399) projected
  line L35 (-5.3633, -11.4634) -> (-5.5062, -11.0504) projected
  line L36 (-5.1983, -11.8783) -> (-5.3633, -11.4634) projected
  line L37 (-5.0602, -12.1901) -> (-5.1983, -11.8783) projected
  line L38 (-2.9375, -12.5288) -> (-5.0602, -12.1901) projected
  line L39 (-2.7092, -12.2754) -> (-2.9375, -12.5288) projected
  line L40 (-2.4233, -11.9325) -> (-2.7092, -12.2754) projected
  line L41 (-2.159, -11.5843) -> (-2.4233, -11.9325) projected
  line L42 (-1.9171, -11.2317) -> (-2.159, -11.5843) projected
  line L43 (-1.6983, -10.8752) -> (-1.9171, -11.2317) projected
  line L44 (-1.5039, -10.5156) -> (-1.6983, -10.8752) projected
  line L45 (-1.3353, -10.1535) -> (-1.5039, -10.5156) projected
  line L46 (-1.1949, -9.7897) -> (-1.3353, -10.1535) projected
  line L47 (-1.0869, -9.4249) -> (-1.1949, -9.7897) projected
  line L48 (-1.0212, -9.0599) -> (-1.0869, -9.4249) projected
  line L49 (-1.0187, -8.6955) -> (-1.0212, -9.0599) projected
  line L50 (-0.9863, -8.3307) -> (-1.0187, -8.6955) projected
  line L51 (-0.9519, -8.1479) -> (-0.9863, -8.3307) projected
  line L52 (-0.9024, -7.9646) -> (-0.9519, -8.1479) projected
  line L53 (-0.834, -7.7806) -> (-0.9024, -7.9646) projected
  line L54 (-0.74, -7.5953) -> (-0.834, -7.7806) projected
  line L55 (-0.6795, -7.5017) -> (-0.74, -7.5953) projected
  line L56 (-0.6059, -7.4072) -> (-0.6795, -7.5017) projected
  line L57 (-0.5127, -7.3112) -> (-0.6059, -7.4072) projected
  line L58 (-0.3829, -7.2119) -> (-0.5127, -7.3112) projected
  line L59 (-0.0429, -7.0929) -> (-0.3829, -7.2119) projected
  line L60 (0.6951, -6.9997) -> (-0.0429, -7.0929) projected
  line L61 (1.4262, -6.8619) -> (0.6951, -6.9997) projected
  line L62 (1.7863, -6.8709) -> (1.4262, -6.8619) projected
  line L63 (1.9402, -6.9255) -> (1.7863, -6.8709) projected
  line L64 (2.0585, -6.9883) -> (1.9402, -6.9255) projected
  line L65 (2.1575, -7.0556) -> (2.0585, -6.9883) projected
  line L66 (2.2438, -7.1261) -> (2.1575, -7.0556) projected
  line L67 (2.3901, -7.2737) -> (2.2438, -7.1261) projected
  line L68 (2.5117, -7.4278) -> (2.3901, -7.2737) projected
  line L69 (2.615, -7.5871) -> (2.5117, -7.4278) projected
  line L70 (2.7039, -7.7505) -> (2.615, -7.5871) projected
  line L71 (2.8467, -8.0877) -> (2.7039, -7.7505) projected
  line L72 (2.9609, -8.4338) -> (2.8467, -8.0877) projected
  line L73 (3.1354, -8.7611) -> (2.9609, -8.4338) projected
  line L74 (3.3502, -9.0751) -> (3.1354, -8.7611) projected
  line L75 (3.5955, -9.3782) -> (3.3502, -9.0751) projected
  line L76 (3.867, -9.6711) -> (3.5955, -9.3782) projected
  line L77 (4.1624, -9.9537) -> (3.867, -9.6711) projected
  line L78 (4.48, -10.2258) -> (4.1624, -9.9537) projected
  line L79 (4.8185, -10.4872) -> (4.48, -10.2258) projected
  line L80 (5.1768, -10.7375) -> (4.8185, -10.4872) projected
  line L81 (5.5542, -10.9761) -> (5.1768, -10.7375) projected
  line L82 (5.8492, -11.1472) -> (5.5542, -10.9761) projected
  line L83 (7.7656, -10.1735) -> (5.8492, -11.1472) projected
  line L84 (7.8013, -9.8343) -> (7.7656, -10.1735) projected
  line L85 (7.8311, -9.3888) -> (7.8013, -9.8343) projected
  line L86 (7.8403, -8.9518) -> (7.8311, -9.3888) projected
  line L87 (7.8287, -8.5243) -> (7.8403, -8.9518) projected
  line L88 (7.7961, -8.1074) -> (7.8287, -8.5243) projected
  line L89 (7.742, -7.7022) -> (7.7961, -8.1074) projected
  line L90 (7.6656, -7.3102) -> (7.742, -7.7022) projected
  line L91 (7.5654, -6.9333) -> (7.6656, -7.3102) projected
  line L92 (7.4384, -6.5746) -> (7.5654, -6.9333) projected
  line L93 (7.2769, -6.2407) -> (7.4384, -6.5746) projected
  line L94 (7.0647, -5.9445) -> (7.2769, -6.2407) projected
  line L95 (6.8765, -5.6303) -> (7.0647, -5.9445) projected
  line L96 (6.7969, -5.4622) -> (6.8765, -5.6303) projected
  line L97 (6.7292, -5.2848) -> (6.7969, -5.4622) projected
  line L98 (6.6764, -5.0958) -> (6.7292, -5.2848) projected
  line L99 (6.6435, -4.8906) -> (6.6764, -5.0958) projected
  line L100 (6.6374, -4.7793) -> (6.6435, -4.8906) projected
  line L101 (6.6415, -4.6596) -> (6.6374, -4.7793) projected
  line L102 (6.6604, -4.5271) -> (6.6415, -4.6596) projected
  line L103 (6.7071, -4.3705) -> (6.6604, -4.5271) projected
  line L104 (6.9122, -4.0744) -> (6.7071, -4.3705) projected
  line L105 (7.4545, -3.5652) -> (6.9122, -4.0744) projected
  line L106 (7.9649, -3.024) -> (7.4545, -3.5652) projected
  line L107 (8.2615, -2.8196) -> (7.9649, -3.024) projected
  line L108 (8.4182, -2.7733) -> (8.2615, -2.8196) projected
  line L109 (8.5508, -2.7546) -> (8.4182, -2.7733) projected
  line L110 (8.6705, -2.7509) -> (8.5508, -2.7546) projected
  line L111 (8.7817, -2.7571) -> (8.6705, -2.7509) projected
  line L112 (8.9868, -2.7905) -> (8.7817, -2.7571) projected
  line L113 (9.1758, -2.8438) -> (8.9868, -2.7905) projected
  line L114 (9.353, -2.9118) -> (9.1758, -2.8438) projected
  line L115 (9.5209, -2.9918) -> (9.353, -2.9118) projected
  line L116 (9.8347, -3.1808) -> (9.5209, -2.9918) projected
  line L117 (10.1304, -3.3936) -> (9.8347, -3.1808) projected
  line L118 (10.464, -3.5558) -> (10.1304, -3.3936) projected
  line L119 (10.8224, -3.6836) -> (10.464, -3.5558) projected
  line L120 (11.199, -3.7847) -> (10.8224, -3.6836) projected
  line L121 (11.5908, -3.862) -> (11.199, -3.7847) projected
  line L122 (11.9959, -3.917) -> (11.5908, -3.862) projected
  line L123 (12.4128, -3.9505) -> (11.9959, -3.917) projected
  line L124 (12.8403, -3.963) -> (12.4128, -3.9505) projected
  line L125 (13.2773, -3.9548) -> (12.8403, -3.963) projected
  line L126 (13.7228, -3.9261) -> (13.2773, -3.9548) projected
  line L127 (14.0621, -3.891) -> (13.7228, -3.9261) projected
  line L128 (15.0401, -1.9769) -> (14.0621, -3.891) projected
  line L129 (14.8697, -1.6815) -> (15.0401, -1.9769) projected
  line L130 (14.6319, -1.3036) -> (14.8697, -1.6815) projected
  line L131 (14.3824, -0.9447) -> (14.6319, -1.3036) projected
  line L132 (14.1218, -0.6056) -> (14.3824, -0.9447) projected
  line L133 (13.8504, -0.2874) -> (14.1218, -0.6056) projected
  line L134 (13.5684, 0.0086) -> (13.8504, -0.2874) projected
  line L135 (13.2762, 0.2808) -> (13.5684, 0.0086) projected
  line L136 (12.9736, 0.5268) -> (13.2762, 0.2808) projected
  line L137 (12.66, 0.7423) -> (12.9736, 0.5268) projected
  line L138 (12.3332, 0.9175) -> (12.66, 0.7423) projected
  line L139 (11.9874, 1.0325) -> (12.3332, 0.9175) projected
  line L140 (11.6504, 1.1761) -> (11.9874, 1.0325) projected
  line L141 (11.4872, 1.2653) -> (11.6504, 1.1761) projected
  line L142 (11.3282, 1.369) -> (11.4872, 1.2653) projected
  line L143 (11.1743, 1.4909) -> (11.3282, 1.369) projected
  line L144 (11.0271, 1.6375) -> (11.1743, 1.4909) projected
  line L145 (10.9568, 1.724) -> (11.0271, 1.6375) projected
  line L146 (10.8897, 1.8232) -> (10.9568, 1.724) projected
  line L147 (10.8272, 1.9416) -> (10.8897, 1.8232) projected
  line L148 (10.7729, 2.0956) -> (10.8272, 1.9416) projected
  line L149 (10.7647, 2.4558) -> (10.7729, 2.0956) projected
  line L150 (10.9042, 3.1865) -> (10.7647, 2.4558) projected
  line L151 (10.999, 3.9243) -> (10.9042, 3.1865) projected
  line L152 (11.1188, 4.264) -> (10.999, 3.9243) projected
  line L153 (11.2183, 4.3936) -> (11.1188, 4.264) projected
  line L154 (11.3146, 4.4866) -> (11.2183, 4.3936) projected
  line L155 (11.4093, 4.56) -> (11.3146, 4.4866) projected
  line L156 (11.5029, 4.6203) -> (11.4093, 4.56) projected
  line L157 (11.6885, 4.7139) -> (11.5029, 4.6203) projected
  line L158 (11.8727, 4.7818) -> (11.6885, 4.7139) projected
  line L159 (12.056, 4.8309) -> (11.8727, 4.7818) projected
  line L160 (12.2389, 4.8649) -> (12.056, 4.8309) projected
  line L161 (12.6038, 4.8965) -> (12.2389, 4.8649) projected
  line L162 (12.9682, 4.8982) -> (12.6038, 4.8965) projected
  line L163 (13.3334, 4.963) -> (12.9682, 4.8982) projected
  line L164 (13.6984, 5.0703) -> (13.3334, 4.963) projected
  line L165 (14.0625, 5.2099) -> (13.6984, 5.0703) projected
  line L166 (14.425, 5.3776) -> (14.0625, 5.2099) projected
  line L167 (14.785, 5.5713) -> (14.425, 5.3776) projected
  line L168 (15.142, 5.7892) -> (14.785, 5.5713) projected
  line L169 (15.4952, 6.0303) -> (15.142, 5.7892) projected
  line L170 (15.8439, 6.2938) -> (15.4952, 6.0303) projected
  line L171 (16.1875, 6.579) -> (15.8439, 6.2938) projected
  line L172 (16.4414, 6.8067) -> (16.1875, 6.579) projected
  line L173 (16.1075, 8.9301) -> (16.4414, 6.8067) projected
  line L174 (15.796, 9.069) -> (16.1075, 8.9301) projected
  line L175 (15.3815, 9.2349) -> (15.796, 9.069) projected
  line L176 (14.9687, 9.3787) -> (15.3815, 9.2349) projected
  line L177 (14.5586, 9.4998) -> (14.9687, 9.3787) projected
  line L178 (14.1519, 9.5976) -> (14.5586, 9.4998) projected
  line L179 (13.7498, 9.6714) -> (14.1519, 9.5976) projected
  line L180 (13.3534, 9.7199) -> (13.7498, 9.6714) projected
  line L181 (12.964, 9.741) -> (13.3534, 9.7199) projected
  line L182 (12.5837, 9.731) -> (12.964, 9.741) projected
  line L183 (12.2162, 9.6807) -> (12.5837, 9.731) projected
  line L184 (11.8689, 9.5704) -> (12.2162, 9.6807) projected
  line L185 (11.5119, 9.4885) -> (11.8689, 9.5704) projected
  line L186 (11.3274, 9.4648) -> (11.5119, 9.4885) projected
  line L187 (11.1379, 9.4552) -> (11.3274, 9.4648) projected
  line L188 (10.9417, 9.4634) -> (11.1379, 9.4552) projected
  line L189 (10.7364, 9.4955) -> (10.9417, 9.4634) projected
  line L190 (10.6287, 9.5241) -> (10.7364, 9.4955) projected
  line L191 (10.5161, 9.5649) -> (10.6287, 9.5241) projected
  line L192 (10.3959, 9.6239) -> (10.5161, 9.5649) projected
  line L193 (10.2615, 9.7167) -> (10.3959, 9.6239) projected
  line L194 (10.0432, 10.0032) -> (10.2615, 9.7167) projected
  line L195 (9.7265, 10.6764) -> (10.0432, 10.0032) projected
  line L196 (9.3696, 11.329) -> (9.7265, 10.6764) projected
  line L197 (9.2668, 11.6743) -> (9.3696, 11.329) projected
  line L198 (9.2712, 11.8376) -> (9.2668, 11.6743) projected
  line L199 (9.2943, 11.9695) -> (9.2712, 11.8376) projected
  line L200 (9.3278, 12.0845) -> (9.2943, 11.9695) projected
  line L201 (9.3681, 12.1883) -> (9.3278, 12.0845) projected
  line L202 (9.4633, 12.3731) -> (9.3681, 12.1883) projected
  line L203 (9.5723, 12.5363) -> (9.4633, 12.3731) projected
  line L204 (9.6918, 12.6838) -> (9.5723, 12.5363) projected
  line L205 (9.8198, 12.8188) -> (9.6918, 12.6838) projected
  line L206 (10.0964, 13.0589) -> (9.8198, 12.8188) projected
  line L207 (10.3902, 13.2744) -> (10.0964, 13.0589) projected
  line L208 (10.6476, 13.5415) -> (10.3902, 13.2744) projected
  line L209 (10.8798, 13.8428) -> (10.6476, 13.5415) projected
  line L210 (11.0924, 14.1698) -> (10.8798, 13.8428) projected
  circle A2 centre (-8.3767, 1.5633) radius 1.6 projected
  circle A3 centre (2.3455, -2.0471) radius 1.6 projected
  circle A4 centre (5.9559, 8.675) radius 1.6 projected
  circle A5 centre (-4.7663, 12.2855) radius 1.6 projected
  circle A6 centre (-1.2104, 5.1192) radius 2.5 projected
  point P0 (0, 0)
  dimension "d4" = 30
  dimension "d5" = 30
  dimension "d6" = 4
  constraints: 10 end point, 2 perpendicular, 1 parallel, 1 point on line
  measures "d4" distance of L0.start L1.end
  measures "d5" distance of L1.end L2.end
  measures "d6" distance of L2.end L3.end
extrude "Выдавливание3" add sketch "Эскиз3" against normal up to surface (5 mm away) contours L0 L5 L4 L3 L2 L1
sketch "Эскиз4" plane through (0, 0, 0) normal (0, 0, -1) x (-1, 0, 0)
  line L0 (11.1891, 14.3431) -> (11.0924, 14.1698) projected
  arc A0 (11.1891, 14.3431) -> (-16.1963, 14.3431) centre (-2.5036, -3.8906) ccw projected
  arc A1 (-25.3405, 9.161) -> (-16.1963, 14.3431) centre (-40.8164, 47.1281) ccw projected
  line L1 (-25.3405, 9.161) -> (-53, 20.778) projected
  line L2 (-53, 20.778) -> (-76.2555, 1.8259) projected
  line L3 (-76.2555, 1.8259) -> (-73.7286, -1.2748) projected
  line L4 (-73.7286, -1.2748) -> (-53, 15.6179) projected
  line L5 (-53, 15.6179) -> (-25.3405, 4.0009) projected
  line L6 (-25.3405, 4.0009) -> (-25.3405, -5.5092) projected
  line L7 (-25.3405, -5.5092) -> (-8.4316, -5.5092) projected
  line L8 (-8.3032, -5.4435) -> (-8.4316, -5.5092) projected
  line L9 (-8.1993, -5.4034) -> (-8.3032, -5.4435) projected
  line L10 (-8.0842, -5.3702) -> (-8.1993, -5.4034) projected
  line L11 (-7.9523, -5.3473) -> (-8.0842, -5.3702) projected
  line L12 (-7.789, -5.3433) -> (-7.9523, -5.3473) projected
  line L13 (-7.444, -5.4468) -> (-7.789, -5.3433) projected
  line L14 (-6.7921, -5.8052) -> (-7.444, -5.4468) projected
  line L15 (-6.1197, -6.1235) -> (-6.7921, -5.8052) projected
  line L16 (-5.8336, -6.3424) -> (-6.1197, -6.1235) projected
  line L17 (-5.7412, -6.4771) -> (-5.8336, -6.3424) projected
  line L18 (-5.6824, -6.5974) -> (-5.7412, -6.4771) projected
  line L19 (-5.6419, -6.7101) -> (-5.6824, -6.5974) projected
  line L20 (-5.6135, -6.8178) -> (-5.6419, -6.7101) projected
  line L21 (-5.5818, -7.0232) -> (-5.6135, -6.8178) projected
  line L22 (-5.5741, -7.2193) -> (-5.5818, -7.0232) projected
  line L23 (-5.5841, -7.4089) -> (-5.5741, -7.2193) projected
  line L24 (-5.6083, -7.5933) -> (-5.5841, -7.4089) projected
  line L25 (-5.691, -7.9502) -> (-5.6083, -7.5933) projected
  line L26 (-5.802, -8.2972) -> (-5.691, -7.9502) projected
  line L27 (-5.8532, -8.6645) -> (-5.802, -8.2972) projected
  line L28 (-5.864, -9.0449) -> (-5.8532, -8.6645) projected
  line L29 (-5.8437, -9.4343) -> (-5.864, -9.0449) projected
  line L30 (-5.7962, -9.8308) -> (-5.8437, -9.4343) projected
  line L31 (-5.7233, -10.2331) -> (-5.7962, -9.8308) projected
  line L32 (-5.6263, -10.6399) -> (-5.7233, -10.2331) projected
  line L33 (-5.5062, -11.0504) -> (-5.6263, -10.6399) projected
  line L34 (-5.3633, -11.4634) -> (-5.5062, -11.0504) projected
  line L35 (-5.1983, -11.8783) -> (-5.3633, -11.4634) projected
  line L36 (-5.0602, -12.1901) -> (-5.1983, -11.8783) projected
  line L37 (-2.9375, -12.5288) -> (-5.0602, -12.1901) projected
  line L38 (-2.7092, -12.2754) -> (-2.9375, -12.5288) projected
  line L39 (-2.4233, -11.9325) -> (-2.7092, -12.2754) projected
  line L40 (-2.159, -11.5843) -> (-2.4233, -11.9325) projected
  line L41 (-1.9171, -11.2317) -> (-2.159, -11.5843) projected
  line L42 (-1.6983, -10.8752) -> (-1.9171, -11.2317) projected
  line L43 (-1.5039, -10.5156) -> (-1.6983, -10.8752) projected
  line L44 (-1.3353, -10.1535) -> (-1.5039, -10.5156) projected
  line L45 (-1.1949, -9.7897) -> (-1.3353, -10.1535) projected
  line L46 (-1.0869, -9.4249) -> (-1.1949, -9.7897) projected
  line L47 (-1.0212, -9.0599) -> (-1.0869, -9.4249) projected
  line L48 (-1.0187, -8.6955) -> (-1.0212, -9.0599) projected
  line L49 (-0.9863, -8.3307) -> (-1.0187, -8.6955) projected
  line L50 (-0.9519, -8.1479) -> (-0.9863, -8.3307) projected
  line L51 (-0.9024, -7.9646) -> (-0.9519, -8.1479) projected
  line L52 (-0.834, -7.7806) -> (-0.9024, -7.9646) projected
  line L53 (-0.74, -7.5953) -> (-0.834, -7.7806) projected
  line L54 (-0.6795, -7.5017) -> (-0.74, -7.5953) projected
  line L55 (-0.6059, -7.4072) -> (-0.6795, -7.5017) projected
  line L56 (-0.5127, -7.3112) -> (-0.6059, -7.4072) projected
  line L57 (-0.3829, -7.2119) -> (-0.5127, -7.3112) projected
  line L58 (-0.0429, -7.0929) -> (-0.3829, -7.2119) projected
  line L59 (0.6951, -6.9997) -> (-0.0429, -7.0929) projected
  line L60 (1.4262, -6.8619) -> (0.6951, -6.9997) projected
  line L61 (1.7863, -6.8709) -> (1.4262, -6.8619) projected
  line L62 (1.9402, -6.9255) -> (1.7863, -6.8709) projected
  line L63 (2.0585, -6.9883) -> (1.9402, -6.9255) projected
  line L64 (2.1575, -7.0556) -> (2.0585, -6.9883) projected
  line L65 (2.2438, -7.1261) -> (2.1575, -7.0556) projected
  line L66 (2.3901, -7.2737) -> (2.2438, -7.1261) projected
  line L67 (2.5117, -7.4278) -> (2.3901, -7.2737) projected
  line L68 (2.615, -7.5871) -> (2.5117, -7.4278) projected
  line L69 (2.7039, -7.7505) -> (2.615, -7.5871) projected
  line L70 (2.8467, -8.0877) -> (2.7039, -7.7505) projected
  line L71 (2.9609, -8.4338) -> (2.8467, -8.0877) projected
  line L72 (3.1354, -8.7611) -> (2.9609, -8.4338) projected
  line L73 (3.3502, -9.0751) -> (3.1354, -8.7611) projected
  line L74 (3.5955, -9.3782) -> (3.3502, -9.0751) projected
  line L75 (3.867, -9.6711) -> (3.5955, -9.3782) projected
  line L76 (4.1624, -9.9537) -> (3.867, -9.6711) projected
  line L77 (4.48, -10.2258) -> (4.1624, -9.9537) projected
  line L78 (4.8185, -10.4872) -> (4.48, -10.2258) projected
  line L79 (5.1768, -10.7375) -> (4.8185, -10.4872) projected
  line L80 (5.5542, -10.9761) -> (5.1768, -10.7375) projected
  line L81 (5.8492, -11.1472) -> (5.5542, -10.9761) projected
  line L82 (7.7656, -10.1735) -> (5.8492, -11.1472) projected
  line L83 (7.8013, -9.8343) -> (7.7656, -10.1735) projected
  line L84 (7.8311, -9.3888) -> (7.8013, -9.8343) projected
  line L85 (7.8403, -8.9518) -> (7.8311, -9.3888) projected
  line L86 (7.8287, -8.5243) -> (7.8403, -8.9518) projected
  line L87 (7.7961, -8.1074) -> (7.8287, -8.5243) projected
  line L88 (7.742, -7.7022) -> (7.7961, -8.1074) projected
  line L89 (7.6656, -7.3102) -> (7.742, -7.7022) projected
  line L90 (7.5654, -6.9333) -> (7.6656, -7.3102) projected
  line L91 (7.4384, -6.5746) -> (7.5654, -6.9333) projected
  line L92 (7.2769, -6.2407) -> (7.4384, -6.5746) projected
  line L93 (7.0647, -5.9445) -> (7.2769, -6.2407) projected
  line L94 (6.8765, -5.6303) -> (7.0647, -5.9445) projected
  line L95 (6.7969, -5.4622) -> (6.8765, -5.6303) projected
  line L96 (6.7292, -5.2848) -> (6.7969, -5.4622) projected
  line L97 (6.6764, -5.0958) -> (6.7292, -5.2848) projected
  line L98 (6.6435, -4.8906) -> (6.6764, -5.0958) projected
  line L99 (6.6374, -4.7793) -> (6.6435, -4.8906) projected
  line L100 (6.6415, -4.6596) -> (6.6374, -4.7793) projected
  line L101 (6.6604, -4.5271) -> (6.6415, -4.6596) projected
  line L102 (6.7071, -4.3705) -> (6.6604, -4.5271) projected
  line L103 (6.9122, -4.0744) -> (6.7071, -4.3705) projected
  line L104 (7.4545, -3.5652) -> (6.9122, -4.0744) projected
  line L105 (7.9649, -3.024) -> (7.4545, -3.5652) projected
  line L106 (8.2615, -2.8196) -> (7.9649, -3.024) projected
  line L107 (8.4182, -2.7733) -> (8.2615, -2.8196) projected
  line L108 (8.5508, -2.7546) -> (8.4182, -2.7733) projected
  line L109 (8.6705, -2.7509) -> (8.5508, -2.7546) projected
  line L110 (8.7817, -2.7571) -> (8.6705, -2.7509) projected
  line L111 (8.9868, -2.7905) -> (8.7817, -2.7571) projected
  line L112 (9.1758, -2.8438) -> (8.9868, -2.7905) projected
  line L113 (9.353, -2.9118) -> (9.1758, -2.8438) projected
  line L114 (9.5209, -2.9918) -> (9.353, -2.9118) projected
  line L115 (9.8347, -3.1808) -> (9.5209, -2.9918) projected
  line L116 (10.1304, -3.3936) -> (9.8347, -3.1808) projected
  line L117 (10.464, -3.5558) -> (10.1304, -3.3936) projected
  line L118 (10.8224, -3.6836) -> (10.464, -3.5558) projected
  line L119 (11.199, -3.7847) -> (10.8224, -3.6836) projected
  line L120 (11.5908, -3.862) -> (11.199, -3.7847) projected
  line L121 (11.9959, -3.917) -> (11.5908, -3.862) projected
  line L122 (12.4128, -3.9505) -> (11.9959, -3.917) projected
  line L123 (12.8403, -3.963) -> (12.4128, -3.9505) projected
  line L124 (13.2773, -3.9548) -> (12.8403, -3.963) projected
  line L125 (13.7228, -3.9261) -> (13.2773, -3.9548) projected
  line L126 (14.0621, -3.891) -> (13.7228, -3.9261) projected
  line L127 (15.0401, -1.9769) -> (14.0621, -3.891) projected
  line L128 (14.8697, -1.6815) -> (15.0401, -1.9769) projected
  line L129 (14.6319, -1.3036) -> (14.8697, -1.6815) projected
  line L130 (14.3824, -0.9447) -> (14.6319, -1.3036) projected
  line L131 (14.1218, -0.6056) -> (14.3824, -0.9447) projected
  line L132 (13.8504, -0.2874) -> (14.1218, -0.6056) projected
  line L133 (13.5684, 0.0086) -> (13.8504, -0.2874) projected
  line L134 (13.2762, 0.2808) -> (13.5684, 0.0086) projected
  line L135 (12.9736, 0.5268) -> (13.2762, 0.2808) projected
  line L136 (12.66, 0.7423) -> (12.9736, 0.5268) projected
  line L137 (12.3332, 0.9175) -> (12.66, 0.7423) projected
  line L138 (11.9874, 1.0325) -> (12.3332, 0.9175) projected
  line L139 (11.6504, 1.1761) -> (11.9874, 1.0325) projected
  line L140 (11.4872, 1.2653) -> (11.6504, 1.1761) projected
  line L141 (11.3282, 1.369) -> (11.4872, 1.2653) projected
  line L142 (11.1743, 1.4909) -> (11.3282, 1.369) projected
  line L143 (11.0271, 1.6375) -> (11.1743, 1.4909) projected
  line L144 (10.9568, 1.724) -> (11.0271, 1.6375) projected
  line L145 (10.8897, 1.8232) -> (10.9568, 1.724) projected
  line L146 (10.8272, 1.9416) -> (10.8897, 1.8232) projected
  line L147 (10.7729, 2.0956) -> (10.8272, 1.9416) projected
  line L148 (10.7647, 2.4558) -> (10.7729, 2.0956) projected
  line L149 (10.9042, 3.1865) -> (10.7647, 2.4558) projected
  line L150 (10.999, 3.9243) -> (10.9042, 3.1865) projected
  line L151 (11.1188, 4.264) -> (10.999, 3.9243) projected
  line L152 (11.2183, 4.3936) -> (11.1188, 4.264) projected
  line L153 (11.3146, 4.4866) -> (11.2183, 4.3936) projected
  line L154 (11.4093, 4.56) -> (11.3146, 4.4866) projected
  line L155 (11.5029, 4.6203) -> (11.4093, 4.56) projected
  line L156 (11.6885, 4.7139) -> (11.5029, 4.6203) projected
  line L157 (11.8727, 4.7818) -> (11.6885, 4.7139) projected
  line L158 (12.056, 4.8309) -> (11.8727, 4.7818) projected
  line L159 (12.2389, 4.8649) -> (12.056, 4.8309) projected
  line L160 (12.6038, 4.8965) -> (12.2389, 4.8649) projected
  line L161 (12.9682, 4.8982) -> (12.6038, 4.8965) projected
  line L162 (13.3334, 4.963) -> (12.9682, 4.8982) projected
  line L163 (13.6984, 5.0703) -> (13.3334, 4.963) projected
  line L164 (14.0625, 5.2099) -> (13.6984, 5.0703) projected
  line L165 (14.425, 5.3776) -> (14.0625, 5.2099) projected
  line L166 (14.785, 5.5713) -> (14.425, 5.3776) projected
  line L167 (15.142, 5.7892) -> (14.785, 5.5713) projected
  line L168 (15.4952, 6.0303) -> (15.142, 5.7892) projected
  line L169 (15.8439, 6.2938) -> (15.4952, 6.0303) projected
  line L170 (16.1875, 6.579) -> (15.8439, 6.2938) projected
  line L171 (16.4414, 6.8067) -> (16.1875, 6.579) projected
  line L172 (16.1075, 8.9301) -> (16.4414, 6.8067) projected
  line L173 (15.796, 9.069) -> (16.1075, 8.9301) projected
  line L174 (15.3815, 9.2349) -> (15.796, 9.069) projected
  line L175 (14.9687, 9.3787) -> (15.3815, 9.2349) projected
  line L176 (14.5586, 9.4998) -> (14.9687, 9.3787) projected
  line L177 (14.1519, 9.5976) -> (14.5586, 9.4998) projected
  line L178 (13.7498, 9.6714) -> (14.1519, 9.5976) projected
  line L179 (13.3534, 9.7199) -> (13.7498, 9.6714) projected
  line L180 (12.964, 9.741) -> (13.3534, 9.7199) projected
  line L181 (12.5837, 9.731) -> (12.964, 9.741) projected
  line L182 (12.2162, 9.6807) -> (12.5837, 9.731) projected
  line L183 (11.8689, 9.5704) -> (12.2162, 9.6807) projected
  line L184 (11.5119, 9.4885) -> (11.8689, 9.5704) projected
  line L185 (11.3274, 9.4648) -> (11.5119, 9.4885) projected
  line L186 (11.1379, 9.4552) -> (11.3274, 9.4648) projected
  line L187 (10.9417, 9.4634) -> (11.1379, 9.4552) projected
  line L188 (10.7364, 9.4955) -> (10.9417, 9.4634) projected
  line L189 (10.6287, 9.5241) -> (10.7364, 9.4955) projected
  line L190 (10.5161, 9.5649) -> (10.6287, 9.5241) projected
  line L191 (10.3959, 9.6239) -> (10.5161, 9.5649) projected
  line L192 (10.2615, 9.7167) -> (10.3959, 9.6239) projected
  line L193 (10.0432, 10.0032) -> (10.2615, 9.7167) projected
  line L194 (9.7265, 10.6764) -> (10.0432, 10.0032) projected
  line L195 (9.3696, 11.329) -> (9.7265, 10.6764) projected
  line L196 (9.2668, 11.6743) -> (9.3696, 11.329) projected
  line L197 (9.2712, 11.8376) -> (9.2668, 11.6743) projected
  line L198 (9.2943, 11.9695) -> (9.2712, 11.8376) projected
  line L199 (9.3278, 12.0845) -> (9.2943, 11.9695) projected
  line L200 (9.3681, 12.1883) -> (9.3278, 12.0845) projected
  line L201 (9.4633, 12.3731) -> (9.3681, 12.1883) projected
  line L202 (9.5723, 12.5363) -> (9.4633, 12.3731) projected
  line L203 (9.6918, 12.6838) -> (9.5723, 12.5363) projected
  line L204 (9.8198, 12.8188) -> (9.6918, 12.6838) projected
  line L205 (10.0964, 13.0589) -> (9.8198, 12.8188) projected
  line L206 (10.3902, 13.2744) -> (10.0964, 13.0589) projected
  line L207 (10.6476, 13.5415) -> (10.3902, 13.2744) projected
  line L208 (10.8798, 13.8428) -> (10.6476, 13.5415) projected
  line L209 (11.0924, 14.1698) -> (10.8798, 13.8428) projected
  circle A2 centre (-8.3767, 1.5633) radius 1.6 projected
  circle A3 centre (2.3455, -2.0471) radius 1.6 projected
  circle A4 centre (5.9559, 8.675) radius 1.6 projected
  circle A5 centre (-4.7663, 12.2855) radius 1.6 projected
  circle A6 centre (-1.2104, 5.1192) radius 2.5 projected
  line L210 (-25.3405, 4.0009) -> (-25.3405, -5.5092) projected
  line L211 (-8.0842, -5.3702) -> (-25.3405, 4.0009)
  point P0 (0, 0)
  constraints: 2 end point
extrude "Выдавливание4" cut sketch "Эскиз4" against normal through all contours L211 L10 L9 L8 L7 L6
sketch "Эскиз5" plane through (0, 0, 0) normal (0, 0, -1) x (-1, 0, 0)
  line L0 (-53, 15.6179) -> (-25.3405, 4.0009) projected
  line L1 (-53, 15.6179) -> (-53, -9)
  line L2 (-53, -9) -> (-57, -9)
  line L3 (-57, -9) -> (-57, 32)
  line L4 (-25.3405, 9.161) -> (-53, 20.778) projected
  line L5 (-53, 20.778) -> (-57, 20.778)
  line L6 (-53, 20.778) -> (-53, 15.6179)
  point P0 (0, 0)
  dimension "d11" = 4
  constraints: 10 end point, 2 perpendicular, 2 vertical, 1 parallel, 1 point on line
  measures "d11" distance of L1.end L2.end
extrude "Выдавливание5" add sketch "Эскиз5" against normal up to surface (5 mm away)